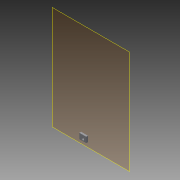
# Autodesk Inventor part: TUNING SPACER
Saved by Autodesk Inventor 2013 (Build 170138000, 138)
## iProperties
Created: 2014-03-07
Part Number: TUNING SPACER
Material: Generic
Document SubType Name: Modeling
Designer: employee
Density: 1 g/cm^3
Author: employee
Autodesk Inventor part; units mm, degrees
ref_plane "YZ Plane" through (0, 0, 0) normal (1, 0, 0) x (0, 1, 0)
ref_plane "XZ Plane" through (0, 0, 0) normal (0, 1, 0) x (-1, 0, 0)
ref_plane "XY Plane" through (0, 0, 0) normal (0, 0, 1) x (1, 0, 0)
ref_plane "Work Plane1" through (0, 0, 0) normal (0, 0, 1) x (1, 0, 0)
sketch "Sketch1" plane through (0, 0, 0) normal (0, 0, 1) x (1, 0, 0)
  circle A0 centre (-140.2575, -162.38) radius 5.08 projected
  circle A1 centre (-132.6242, -154.7468) radius 1.125 projected
  line L0 (-140.2575, -162.38) -> (-140.2575, -149.1787) construction
  circle A2 centre (-147.8907, -154.7468) radius 1.125
  line L1 (-239.2575, -170) -> (4.7425, -170) construction
  line L2 (-152.7575, -150) -> (-127.7575, -150)
  line L3 (-127.7575, -150) -> (-127.7575, -170)
  line L4 (-127.7575, -170) -> (-152.7575, -170)
  line L5 (-152.7575, -170) -> (-152.7575, -150)
  circle A3 centre (-147.8907, -154.7468) radius 0.5
  circle A4 centre (-132.6242, -154.7468) radius 0.5
  point P0 (0, 0)
  point P1 (-140.2575, -170)
  dimension "d0" = 20
  dimension "d2" = 25
  dimension "d3" = 1
  constraints: 10 end point, 2 centre point, 2 coincident, 2 parallel, 1 equal radius, 1 horizontal, 1 midpoint, 1 perpendicular, 1 point on line, 1 symmetric about line, 1 vertical, 1 vertical alignment, 1 other
  measures "d0" distance of L2.end L3.end
  measures "d2" distance of L2.start L2.end
  measures "d3" diameter of A3
extrude "Extrusion1" add sketch "Sketch1" along normal blind 6.477 contours A1 | A2 | L2 L3 L4 L5
fillet "Fillet1" radius 5 4 edges at (-127.7575, -170, 3.2385) (-127.7575, -150, 3.2385) (-152.7575, -170, 3.2385) (-152.7575, -150, 3.2385)
body "Solid1"
